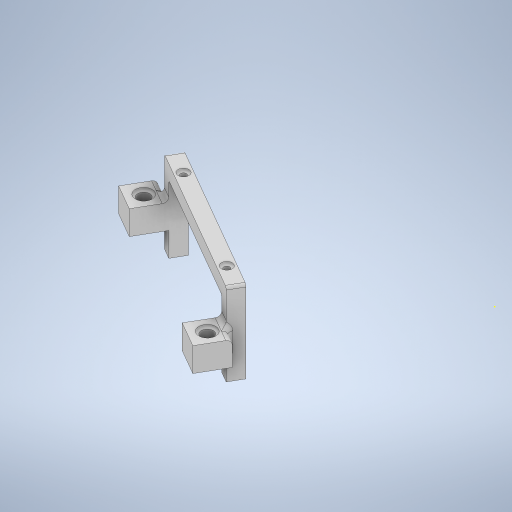
# Autodesk Inventor part: rpimont
Saved by Autodesk Inventor 2023 (Build 270158000, 158)
## iProperties
Created: 2023-11-07
Part Number: rpimont
Material: Ogólny
Document SubType Name: Modeling
Designer: janek
Density: 1 g/cm^3
Appearance: Domyślna
Author: janek
## iProperties of the stored document rpimont_Drukowanie 3D.ipt
Created: 2023-11-13
Part Number: rpimont_Drukowanie 3D
Material: Ogólny
Document SubType Name: Modeling
Designer: janek
Density: 1 g/cm^3
Appearance: Domyślna
Author: janek
Autodesk Inventor part; units mm, degrees
ref_plane "YZ Plane" through (0, 0, 0) normal (1, 0, 0) x (0, 1, 0)
ref_plane "XZ Plane" through (0, 0, 0) normal (0, 1, 0) x (-1, 0, 0)
ref_plane "XY Plane" through (0, 0, 0) normal (0, 0, 1) x (1, 0, 0)
sketch "Szkic1" plane through (0, 0, 0) normal (0, 1, 0) x (-1, 0, 0)
  line L0 (54.3852, -2.6121) -> (97.8852, 72.7321)
  line L1 (54.3852, -2.6121) -> (2.4237, 27.3879)
  line L2 (2.4237, 27.3879) -> (45.9237, 102.7321)
  line L3 (45.9237, 102.7321) -> (97.8852, 72.7321)
  line L4 (0, 133.3679) -> (115.5, 66.684)
  line L5 (32.9237, 80.2155) -> (28.5935, 82.7155)
  line L6 (28.5935, 82.7155) -> (25.5935, 77.5193)
  line L7 (25.5935, 77.5193) -> (29.9237, 75.0193)
  line L8 (84.8852, 50.2155) -> (89.2153, 47.7155)
  line L9 (89.2153, 47.7155) -> (86.2153, 42.5193)
  line L10 (86.2153, 42.5193) -> (81.8852, 45.0193)
  line L11 (28.5935, 82.7155) -> (32.5935, 89.6437)
  line L12 (32.5935, 89.6437) -> (36.9237, 87.1437)
  line L13 (89.2153, 47.7155) -> (93.2153, 54.6437)
  line L14 (93.2153, 54.6437) -> (88.8852, 57.1437)
  line L15 (89.2153, 47.7155) -> (90.9474, 46.7155)
  line L16 (90.9474, 46.7155) -> (94.9474, 53.6437)
  line L17 (94.9474, 53.6437) -> (93.2153, 54.6437)
  line L18 (28.5935, 82.7155) -> (26.8615, 83.7155)
  line L19 (26.8615, 83.7155) -> (30.8615, 90.6437)
  line L20 (30.8615, 90.6437) -> (32.5935, 89.6437)
  line L21 (95.8852, 69.268) -> (108.0096, 62.268)
  line L22 (108.0096, 62.268) -> (97.0096, 43.2155)
  line L23 (97.0096, 43.2155) -> (90.9474, 46.7155)
  line L24 (43.9237, 99.268) -> (31.7993, 106.268)
  line L25 (31.7993, 106.268) -> (20.7993, 87.2155)
  line L26 (20.7993, 87.2155) -> (26.8615, 83.7155)
  line L27 (95.2775, 44.2155) -> (101.2775, 54.6078)
  line L28 (101.2775, 54.6078) -> (90.8852, 60.6078)
  line L29 (28.5314, 96.6078) -> (38.9237, 90.6078)
  line L30 (28.5314, 96.6078) -> (22.5314, 86.2155)
  point P0 (0, 0)
  point P1 (0, 0)
  dimension "d0" = 87
  dimension "d1" = 60
  dimension "d2" = 26
  dimension "d3" = 6
  dimension "d4" = 5
  dimension "d5" = 5
  dimension "d6" = 6
  dimension "d7" = 26
  dimension "d8" = 8
  dimension "d24" = 2
  dimension "d25" = 2
  dimension "d26" = 8
  dimension "d27" = 14
  dimension "d28" = 14
  dimension "d30" = 14
  dimension "d46" = 12
  dimension "d47" = 12
  dimension "d48" = 12
  constraints: 62 end point, 23 perpendicular, 17 point on line, 1 collinear
  measures "d0" distance of L0.start L0.end
  measures "d1" distance of L0.start L1.end
  measures "d2" distance of L2.end L5.start
  measures "d3" distance between parallel lines of L7 L5
  measures "d4" distance between parallel lines of L6 L2
  measures "d5" distance of L8.start L8.end
  measures "d6" distance between parallel lines of L8 L10
  measures "d7" distance of L0.end L8.start
  measures "d8" distance of L5.end L11.end
  measures "d24" distance of L8.end L15.end
  measures "d25" distance of L5.end L18.end
  measures "d26" distance between parallel lines of L14 L8
  measures "d27" distance from line of L14.end L22
  measures "d28" distance between parallel lines of L14 L21
  measures "d30" distance between parallel lines of L25 L2
  measures "d46" distance between parallel lines of L8 L28
  measures "d47" distance between parallel lines of L27 L0
  measures "d48" distance of L29.start L29.end
extrude "Wyciągnięcie proste1" add sketch "Szkic1" along normal blind 34 contours L0 L8 L9 L10 | L7 L6 L5 L2
sketch "Szkic3" plane through (-81.8852, 0, 45.0193) normal (0.8660254, 0, 0.5) x (0.5, 0, -0.8660254)
  line L0 (-6, 34) -> (0, 34) projected
  line L1 (-6, 34) -> (-6, 28)
  line L2 (-6, 0) -> (-6, 34) projected
  line L3 (-6, 28) -> (0, 28)
  line L4 (0, 0) -> (0, 34) projected
  line L5 (0, 34) -> (0, 28)
  line L6 (0, 34) -> (-6, 34)
  point P0 (79.9305, 0)
  point P1 (-6, 8)
  dimension "d13" = 6
  constraints: 8 end point, 3 perpendicular, 2 point on line
  measures "d13" distance of L0.start L1.end
extrude "Wyciągnięcie proste3" add sketch "Szkic3" along normal blind 60
sketch "Szkic4" plane through (0, 34, 0) normal (0, 1, 0) x (1, 0, 0)
  circle A0 centre (-78.6221, -50.3674) radius 1.25
  circle A1 centre (-36.1868, -74.8674) radius 1.25
  line L0 (-86.2153, -42.5193) -> (-89.2153, -47.7155) projected
  line L1 (-89.2153, -47.7155) -> (-28.5935, -82.7155) projected
  line L2 (-25.5935, -77.5193) -> (-86.2153, -42.5193) projected
  point P0 (0, 0)
  dimension "d16" = 2.5
  dimension "d17" = 2.5
  dimension "d18" = 49
  dimension "d19" = 10.5
  dimension "d20" = 3
  dimension "d21" = 3
  constraints: 2 centre point
  measures "d16" diameter of A0
  measures "d17" diameter of A1
  measures "d18" distance of A0.centre A1.centre
  measures "d19" distance from line of L0 A0.centre
  measures "d20" distance from line of L1 A0.centre
  measures "d21" distance from line of L2 A1.centre
extrude "Wyciągnięcie proste4" cut sketch "Szkic4" against normal blind 60
sketch "Szkic5" plane through (0, 0, 0) normal (0, -1, 0) x (1, 0, 0)
  point P0 (0, 0)
extrude "Wyciągnięcie proste5" add sketch "Szkic1" along normal blind 20 contours L0 L14 L13 L8 | L0 L28 L27 L23 L16 L17 L14 | L13 L17 L16 L15 | L5 L11 L12 L2 | L12 L20 L19 L26 L30 L29 L2 | L18 L19 L20 L11
extrude "Wyciągnięcie proste6" cut sketch "Szkic1" along normal blind 10 contours L0 L14 L13 L8 | L13 L17 L16 L15 | L5 L11 L12 L2 | L18 L19 L20 L11
sketch "Szkic7" plane through (0, 20, 0) normal (0, 1, 0) x (1, 0, 0)
  circle A0 centre (-93.0814, -52.4116) radius 2.5
  circle A1 centre (-30.7275, -88.4116) radius 2.5
  line L0 (-32.9237, -80.2155) -> (-38.9237, -90.6078) projected
  line L1 (-95.2775, -44.2155) -> (-101.2775, -54.6078) projected
  line L2 (-89.2153, -47.7155) -> (-95.2775, -44.2155) projected
  line L3 (-38.9237, -90.6078) -> (-28.5314, -96.6078) projected
  point P0 (0, 0)
  dimension "d38" = 5
  dimension "d39" = 5
  dimension "d40" = 6
  dimension "d51" = 6
  dimension "d52" = 6
  dimension "d53" = 6
  constraints: 2 centre point
  measures "d38" diameter of A0
  measures "d39" diameter of A1
  measures "d40" distance from line of L0 A1.centre
  measures "d51" distance from line of L1 A0.centre
  measures "d52" distance from line of L2 A0.centre
  measures "d53" distance from line of L3 A1.centre
extrude "Wyciągnięcie proste7" cut sketch "Szkic7" against normal blind 10
extrude "Wyciągnięcie proste8" cut sketch "Szkic1" along normal blind 10 contours L0 L28 L27 L23 L16 L17 L14 | L12 L20 L19 L26 L30 L29 L2
fillet "Zaokrąglenie1" radius 2 6 edges at (-87.0503, 20, 48.9655) (-89.2153, 15, 47.7155) (-92.2464, 20, 45.9655) (-30.7586, 20, 81.4655) (-28.5935, 15, 82.7155) (-25.5625, 20, 84.4655)
fillet "Zaokrąglenie2" radius 1 4 edges at (-95.5814, 20, 52.4116) (-33.2275, 20, 88.4116) (-79.8721, 34, 50.3674) (-37.4368, 34, 74.8674) inverted yes
fillet "Zaokrąglenie3" radius 1 2 edges at (-31.4237, 28, 77.6174) (-83.3852, 28, 47.6174)
fillet "Zaokrąglenie4" radius 1 2 edges at (-87.7153, 34, 45.1174) (-27.0935, 34, 80.1174)
